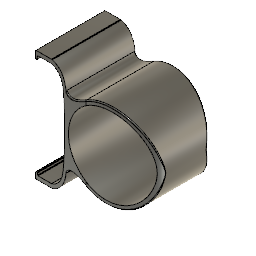
Support Tangon - Anneau (Autodesk Fusion 360 design; units mm, degrees)
Autodesk Fusion 360 part; units mm, degrees
sketch "Sketch3" plane through (0, 0, 0) normal (0, 1, 0) x (1, 0, 0)
  line L0 (2.8008, -105.0675) -> (16.2395, -105.0675)
  spline S0 degree 5 poles (16.2395, -105.0675) (16.5995, -104.9596) (17.3067, -104.7263) (18.3298, -104.3231) (19.6181, -103.6788) (21.0998, -102.6932) (22.4493, -101.5252) (23.6618, -100.1736) (24.7319, -98.64) (25.6544, -96.9294) (26.4267, -95.0509) (27.0504, -93.0181) (27.5339, -90.8504) (27.8945, -88.5741) (28.1555, -86.2193) (28.3432, -83.8176) (28.4839, -81.3992) (28.6017, -78.9906) (28.7145, -76.6114) (28.8341, -74.2735) (28.9671, -71.9836) (29.0867, -70.1922) (29.1842, -68.8718) (29.2528, -68.0018) (29.2879, -67.5693) knots 0 0 0 0 0 0 0.05 0.1 0.15 0.2 0.25 0.3 0.35 0.4 0.45 0.5 0.55 0.6 0.65 0.7 0.75 0.8 0.85 0.9 0.95 1 1 1 1 1 1
  line L1 (-0.001, -106.5675) -> (-0.001, -101.657)
  line L2 (1.8008, -104.0675) -> (1.8008, -101.657)
  line L3 (1.3008, -101.157) -> (0.499, -101.157)
  arc A0 (0.499, -101.157) -> (-0.001, -101.657) centre (0.499, -101.657) ccw
  arc A1 (1.8008, -101.657) -> (1.3008, -101.157) centre (1.3008, -101.657) ccw
  arc A2 (1.8008, -104.0675) -> (2.8008, -105.0675) centre (2.8008, -104.0675) ccw
  line L4 (-6.9477, -107.0334) -> (-6.9477, 2)
  line L5 (-6.9477, -52.5167) -> (73.3246, -52.5167)
  spline S1 degree 5 poles (16.2395, 0.0341) (16.5995, -0.0738) (17.3067, -0.3071) (18.3298, -0.7103) (19.6181, -1.3547) (21.0998, -2.3402) (22.4493, -3.5082) (23.6618, -4.8598) (24.7319, -6.3934) (25.6544, -8.104) (26.4267, -9.9825) (27.0504, -12.0153) (27.5339, -14.183) (27.8945, -16.4593) (28.1555, -18.8141) (28.3432, -21.2158) (28.4839, -23.6342) (28.6017, -26.0428) (28.7145, -28.422) (28.8341, -30.7599) (28.9671, -33.0499) (29.0867, -34.8412) (29.1842, -36.1616) (29.2528, -37.0316) (29.2879, -37.4641) knots 0 0 0 0 0 0 0.05 0.1 0.15 0.2 0.25 0.3 0.35 0.4 0.45 0.5 0.55 0.6 0.65 0.7 0.75 0.8 0.85 0.9 0.95 1 1 1 1 1 1
  line L6 (11.8034, -106.3965) -> (20.6757, -103.7385)
  line L7 (28.9468, -71.7683) -> (29.629, -63.3703)
  line L8 (11.8034, 1.363) -> (20.6757, -1.2949)
  line L9 (28.9468, -33.2651) -> (29.629, -41.6631)
  line L10 (2.8008, 0.0341) -> (16.2395, 0.0341)
  circle A3 centre (73.3246, -52.5167) radius 40
  line L11 (2.8008, -109.0675) -> (16.1173, -109.0675)
  spline S2 degree 3 poles (16.9783, -108.9413) (20.2885, -107.9496) (23.2031, -106.1181) (25.4332, -103.5049) (27.5249, -101.054) (28.9782, -97.9399) (29.8551, -94.5148) (30.9399, -90.2778) (31.2004, -85.6195) (31.4212, -81.226) (31.642, -76.8325) (31.8411, -72.6862) (32.1558, -68.8122) knots 0 0 0 0 0.234827 0.234827 0.234827 0.455076 0.455076 0.455076 0.727538 0.727538 0.727538 1 1 1 1
  spline S3 degree 3 poles (17.0631, 3.8822) (20.3383, 2.8848) (23.2222, 1.0623) (25.4332, -1.5285) (27.5249, -3.9794) (28.9782, -7.0935) (29.8551, -10.5186) (30.9399, -14.7557) (31.2004, -19.414) (31.4212, -23.8075) (31.642, -28.201) (31.8411, -32.3472) (32.1558, -36.2212) knots 0.002009 0.002009 0.002009 0.002009 0.234827 0.234827 0.234827 0.455076 0.455076 0.455076 0.727538 0.727538 0.727538 1 1 1 1
  line L12 (2.8008, 4.0341) -> (16.0435, 4.0341)
  circle A4 centre (73.3246, -52.5167) radius 44
  line L13 (29.2879, -67.5693) -> (29.2879, -37.4641)
  spline S4 degree 5 poles (30.8793, -88.6984) (31.0617, -88.3582) (31.4493, -87.7126) (32.0997, -86.849) (33.1046, -85.9126) (34.5912, -85.1324) (36.3091, -84.7766) (38.2564, -84.8621) (40.4204, -85.3603) (42.7848, -86.2175) (45.3353, -87.3738) (47.5166, -88.4954) (49.2299, -89.4302) (50.4065, -90.0931) (51.0033, -90.4345) knots 0 0 0 0 0 0 0.1 0.2 0.3 0.4 0.5 0.6 0.7 0.8 0.9 1 1 1 1 1 1
  spline S5 degree 5 poles (30.8793, -16.335) (31.0617, -16.6752) (31.4493, -17.3208) (32.0997, -18.1844) (33.1046, -19.1208) (34.5912, -19.901) (36.3091, -20.2568) (38.2564, -20.1713) (40.4204, -19.6731) (42.7848, -18.8159) (45.3353, -17.6596) (47.5166, -16.538) (49.2299, -15.6032) (50.4065, -14.9403) (51.0033, -14.5989) knots 0 0 0 0 0 0 0.1 0.2 0.3 0.4 0.5 0.6 0.7 0.8 0.9 1 1 1 1 1 1
  line L14 (29.7423, -90.8202) -> (32.0164, -86.5766)
  line L15 (48.5135, -89.0104) -> (53.4931, -91.8586)
  line L16 (29.7423, -14.2132) -> (32.0164, -18.4568)
  line L17 (48.5135, -16.023) -> (53.4931, -13.1748)
  line L18 (2.8008, -109.0675) -> (0.379, -109.0675)
  line L19 (-0.001, -108.6875) -> (-0.001, -106.5675)
  arc A5 (-0.001, -108.6875) -> (0.379, -109.0675) centre (0.379, -108.6875) ccw
  arc A6 (16.1173, -109.0675) -> (16.9783, -108.9413) centre (16.1173, -106.0675) ccw
  line L20 (2.8008, 4.0341) -> (0.5, 4.0341)
  line L21 (0, 3.5341) -> (0, -2.4094)
  line L22 (0.5, -2.9094) -> (1.6074, -2.9094)
  line L23 (2.1074, -2.4094) -> (2.1074, -0.4659)
  line L24 (2.6074, 0.0341) -> (7.0857, 0.0341)
  line L25 (5.48, 0.0341) -> (6.6327, 0.0341)
  arc A7 (1.6074, -2.9094) -> (2.1074, -2.4094) centre (1.6074, -2.4094) ccw
  arc A8 (0, -2.4094) -> (0.5, -2.9094) centre (0.5, -2.4094) ccw
  arc A9 (0.5, 4.0341) -> (0, 3.5341) centre (0.5, 3.5341) ccw
  arc A10 (2.6074, 0.0341) -> (2.1074, -0.4659) centre (2.6074, -0.4659) ccw
  arc A11 (17.0631, 3.8822) -> (16.0435, 4.0341) centre (16.0435, 0.5341) ccw
  point P0 (22.8318, -101.0519)
  point P1 (27.0239, -92.9525)
  point P2 (28.5477, -80.065)
  point P3 (3.2913, 2)
  point P4 (22.8318, -3.9815)
  point P5 (27.0239, -12.0809)
  point P6 (28.5477, -24.9684)
  point P7 (36.52, -84.8767)
  point P8 (36.52, -20.1567)
  point P9 (2.1074, 0.0341)
  dimension "d18" = 0.5
  dimension "d19" = 0.5
  dimension "d20" = 1
  dimension "d25" = 80
  dimension "d27" = 4
  dimension "d28" = 0.38
  dimension "d29" = 3
  dimension "d30" = 4.9783
  dimension "d31" = 0.5
  dimension "d32" = 0.5
  dimension "d33" = 0.5
  dimension "d34" = 0.5
  dimension "d35" = 3.5
  constraint horizontal L0
  constraint perpendicular L0 L2
  constraint perpendicular L1 L3
  constraint tangent L1 A0
  constraint tangent L3 A0
  constraint tangent L2 A1
  constraint tangent L3 A1
  constraint tangent L0 A2
  constraint tangent L2 A2
  constraint midpoint L4 L5.start
  constraint perpendicular L4 L5
  constraint midpoint L0.end L6
  constraint midpoint S0.end L7
  constraint symmetric L0.end L5 S1.start
  constraint symmetric P0 L5 P4
  constraint symmetric P1 L5 P5
  constraint symmetric P2 L5 P6
  constraint symmetric S0.end L5 S1.end
  constraint symmetric L0.start L5 L10.start
  constraint symmetric L5 L6.start L8.start
  constraint symmetric L5 L6.end L8.end
  constraint symmetric L5 L7.start L9.start
  constraint symmetric L5 L7.end L9.end
  constraint coincident L5.end A3.centre
  constraint symmetric L5 L11.start L12.start
  constraint symmetric L5 S2.end S3.end
  constraint vertical L13
  constraint coincident S2 S4.start
  constraint coincident A4 S4.end
  constraint midpoint S4.start L14
  constraint midpoint S4.end L15
  constraint symmetric L5 S4.start S5.start
  constraint symmetric L5 P7 P8
  constraint symmetric L5 S4.end S5.end
  constraint symmetric L5 L14.start L16.start
  constraint symmetric L5 L14.end L16.end
  constraint symmetric L5 L15.start L17.start
  constraint symmetric L5 L15.end L17.end
  constraint perpendicular L1 L18
  constraint perpendicular L18 L19
  constraint tangent L18 A5
  constraint tangent L19 A5
  constraint parallel L0 L11
  constraint tangent L11 A6
  constraint tangent S2 A6
  constraint parallel L12 L20
  constraint perpendicular L20 L21
  constraint perpendicular L21 L22
  constraint perpendicular L10 L23
  constraint perpendicular L23 L24
  constraint perpendicular L13 L25
  constraint tangent L22 A7
  constraint tangent L23 A7
  constraint tangent L21 A8
  constraint tangent L22 A8
  constraint tangent L20 A9
  constraint tangent L21 A9
  constraint coincident P9 L23
  constraint coincident P9 L24
  constraint tangent L23 A10
  constraint tangent L24 A10
  constraint tangent S3 A11
  constraint tangent L12 A11
  measures "d18" radius of A0
  measures "d19" radius of A1
  measures "d20" radius of A2
  measures "d25" diameter of A3
  measures "d28" radius of A5
  measures "d29" radius of A6
  measures "d30" distance of P9 L24.end
  measures "d31" radius of A7
  measures "d32" radius of A8
  measures "d33" radius of A9
  measures "d34" radius of A10
  measures "d35" radius of A11
extrude "Extrude3" add sketch "Sketch3" along normal blind 70
sketch "Sketch7" plane through (0, 0, 0) normal (0, 0, 1) x (1, 0, 0)
  line L0 (117.3246, 0) -> (51.0033, 0)
  line L1 (51.0033, 0) -> (51.0033, 70)
  line L2 (117.3246, 70) -> (51.0033, 70)
  line L3 (51.0033, 70) -> (51.0033, 0)
  line L4 (51.0033, 0) -> (117.3246, 15.5097)
  line L5 (51.0033, 35) -> (117.3246, 35)
  spline S0 degree 5 poles (117.3246, 15.5097) (117.4658, 14.5453) (117.0784, 12.6564) (114.4897, 9.9429) (107.4566, 6.5816) (93.8426, 3.0168) (79.336, 0.9954) (66.1546, 0.1811) (56.2415, 0) (51.0033, 0) knots 0 0 0 0 0 0 0.2 0.4 0.6 0.8 1 1 1 1 1 1
  line L6 (63.9682, 0) -> (38.0384, 0)
  line L7 (117.3246, 15.5097) -> (117.3246, 0)
  spline S1 degree 5 poles (117.3246, 54.4903) (117.4658, 55.4547) (117.0784, 57.3436) (114.4897, 60.0571) (107.4566, 63.4184) (93.8426, 66.9832) (79.336, 69.0046) (66.1546, 69.8189) (56.2415, 70) (51.0033, 70) knots 0 0 0 0 0 0 0.2 0.4 0.6 0.8 1 1 1 1 1 1
  line L8 (117.0817, 17.1686) -> (117.5675, 13.8508)
  line L9 (117.0817, 52.8314) -> (117.5675, 56.1492)
  line L10 (63.9682, 70) -> (38.0384, 70)
  line L11 (117.3246, 70) -> (51.0033, 70)
  line L12 (117.3246, 54.4903) -> (117.3246, 70)
  constraint coincident L0.end L1.start
  constraint midpoint L1 L5.start
  constraint perpendicular L1 L5
  constraint midpoint L0.end L6
  constraint coincident L0 L6.start
  constraint coincident L0.start L7.end
  constraint perpendicular L0 L7
  constraint midpoint L4.end L8
  constraint symmetric L0.start L5 L2.start
  constraint symmetric L0.end L5 L1.end
  constraint symmetric L4.end L5 S1.start
  constraint symmetric L5 L0.end L1.end
  constraint symmetric L5 L6.start L10.start
  constraint symmetric L5 L6.end L10.end
  constraint symmetric L5 L0.start L2.start
  constraint symmetric L5 L8.start L9.start
  constraint symmetric L5 L8.end L9.end
extrude "Extrude6" cut sketch "Sketch7" along normal through all contours L0 S0 L6 L7 | L2 S1 L10 L11 L12
fillet "Fillet1" radius 1 4 edges at (96.2423, 3.9975, 90.077) (97.0785, 4.1837, 15.4796) (38.3106, 0, 84.965) (38.3106, 0, 20.0684)
fillet "Fillet2" radius 1 4 edges at (38.3106, 70, 84.965) (96.2486, 66.0011, 14.9603) (97.0877, 65.8143, 89.548) (38.3106, 70, 20.0684)
